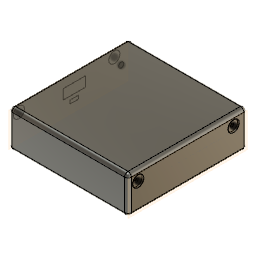
Pedant_lijunchen (Autodesk Fusion 360 design; units mm, degrees)
Autodesk Fusion 360 part; units mm, degrees
sketch "Sketch1" plane through (0, 0, 0) normal (0, 1, 0) x (1, 0, 0) in component "Case"
  line L0 (-35, -10) -> (35, -10)
  line L1 (35, -10) -> (35, 10)
  line L2 (35, 10) -> (-35, 10)
  line L3 (-35, 10) -> (-35, -10)
  dimension "d1" = 70
  dimension "d2" = 20
  dimension "d4" = 35
  dimension "d5" = 10
  constraint horizontal L0
  constraint vertical L1
  constraint horizontal L2
  constraint vertical L3
  measures "d1" distance of L0.start L0.end
  measures "d2" distance of L0.start L2.end
  measures "d4" horizontal distance of origin L0.start
  measures "d5" vertical distance of origin L0.start
extrude "Extrude1" add sketch "Sketch1" along normal blind 70 makes body 1 in component "Case"
shell "Shell1" thickness 2 removed faces 1 at (-11.6667, 23.3333, 10) on bodies 1 in component "Case"
sketch "Sketch2" plane through (-35, 0, 0) normal (-1, 0, 0) x (0, -1, 0) in component "Case"
  line L0 (0, -10) -> (0, 10)
  line L1 (0, 10) -> (-70, 10)
  line L2 (-70, 10) -> (-70, -10)
  line L3 (-70, -10) -> (0, -10)
  circle A0 centre (-66, 0) radius 1.5
  circle A1 centre (-6, 6) radius 3.25
  circle A2 centre (-62, 6) radius 3.25
  line L4 (-45, 5) -> (-32, 5)
  line L5 (-32, 5) -> (-32, -0.8)
  line L6 (-32, -0.8) -> (-45, -0.8)
  line L7 (-45, -0.8) -> (-45, 5)
  line L8 (-41, -2.8) -> (-36, -2.8)
  line L9 (-36, -2.8) -> (-36, -4.8)
  line L10 (-36, -4.8) -> (-41, -4.8)
  line L11 (-41, -4.8) -> (-41, -2.8)
  dimension "d9" = 3
  dimension "d10" = 4
  dimension "d11" = 10
  dimension "d12" = 6.5
  dimension "d14" = 6
  dimension "d15" = 6.5
  dimension "d16" = 8
  dimension "d17" = 4
  dimension "d29" = 13
  dimension "d30" = 5.8
  dimension "d31" = 5
  dimension "d32" = 2
  dimension "d33" = 5
  dimension "d34" = 25
  dimension "d35" = 2
  dimension "d36" = 4
  dimension "d87" = 4
  constraint horizontal L4
  constraint vertical L5
  constraint horizontal L6
  constraint vertical L7
  constraint horizontal L8
  constraint vertical L9
  constraint horizontal L10
  constraint vertical L11
  measures "d9" diameter of A0
  measures "d10" horizontal distance of L1.end A0.centre
  measures "d11" vertical distance of L1.end A0.centre
  measures "d12" diameter of A1
  measures "d14" horizontal distance of L0.end A1.centre
  measures "d15" diameter of A2
  measures "d16" horizontal distance of L1.end A2.centre
  measures "d17" vertical distance of L1.end A2.centre
  measures "d29" distance of L4.start L4.end
  measures "d30" distance of L4.start L6.end
  measures "d31" distance of L8.start L8.end
  measures "d32" distance of L8.start L10.end
  measures "d33" distance of L1 L4.start
  measures "d34" horizontal distance of L1.end L4.start
  measures "d35" vertical distance of L6.end L8.start
  measures "d36" horizontal distance of L6.end L8.start
  measures "d87" vertical distance of L0.end A1.centre
hole "Hole2" at (-35, 6, 6) direction (1, 0, 0) diameter 2 depth 6 tip angle 118 bodies 1 in component "Case"
hole "Hole1" at (-35, 62, 6) direction (1, 0, 0) diameter 2 depth 6 tip angle 118 bodies 1 in component "Case"
extrude "Extrude2" cut sketch "Sketch2" against normal blind 1 contours A1 | A2 bodies 1 in component "Case"
extrude "Extrude3" cut sketch "Sketch2" against normal blind 6 contours A0 | L4 L5 L6 L7 | L8 L9 L10 L11 bodies 1 in component "Case"
sketch "Sketch3" plane through (0, 70, 0) normal (0, 1, 0) x (-1, 0, 0) in component "Case"
  line L0 (35, -10) -> (35, 10)
  line L1 (35, 10) -> (-35, 10)
  line L2 (-35, 10) -> (-35, -10)
  line L3 (-35, -10) -> (35, -10)
  circle A0 centre (31, 0) radius 1.5
  point P0 (35, 10)
  dimension "d39" = 3
  dimension "d40" = 4
  dimension "d41" = 10
  measures "d39" diameter of A0
  measures "d40" horizontal distance of A0.centre P0
  measures "d41" vertical distance of A0.centre P0
extrude "Extrude4" cut sketch "Sketch3" against normal blind 6 contours A0 bodies 1 in component "Case"
sketch "Sketch4" plane through (35, 0, 0) normal (1, 0, 0) x (0, 1, 0) in component "Case"
  line L0 (0, 10) -> (0, -10)
  line L1 (0, -10) -> (70, -10)
  line L2 (70, -10) -> (70, 10)
  line L3 (70, 10) -> (0, 10)
  circle A0 centre (6, 6) radius 3.25
  circle A1 centre (62, 6) radius 3.25
  dimension "d44" = 6.5
  dimension "d45" = 6
  dimension "d46" = 4
  dimension "d47" = 6.5
  dimension "d48" = 8
  dimension "d49" = 4
  measures "d44" diameter of A0
  measures "d45" horizontal distance of L0.start A0.centre
  measures "d46" vertical distance of L0.start A0.centre
  measures "d47" diameter of A1
  measures "d48" horizontal distance of L2.end A1.centre
  measures "d49" vertical distance of L2.end A1.centre
hole "Hole5" at (35, 62, 6) direction (-1, 0, 0) diameter 2 depth 6 tip angle 118 bodies 1 in component "Case"
hole "Hole4" at (35, 6, 6) direction (-1, 0, 0) diameter 2 depth 6 tip angle 118 bodies 1 in component "Case"
extrude "Extrude5" cut sketch "Sketch4" against normal blind 1 contours A0 | A1 bodies 1 in component "Case"
fillet "Fillet1" radius 2 8 edges at (35, 0, 0) (0, 0, -10) (-35, 0, 0) (35, 70, 0) (0, 70, -10) (-35, 70, 0) (-35, 35, -10) (35, 35, -10) on bodies 1 in component "Case"
sketch "Sketch1 (2)" plane through (0, 0, 10) normal (0, 0, 1) x (-1, 0, 0) in component "Top"
  arc A0 (-33, 0) -> (-35, -2) centre (-33, -2) ccw
  line L0 (-35, -2) -> (-35, -68)
  arc A1 (-35, -68) -> (-33, -70) centre (-33, -68) ccw
  line L1 (-33, -70) -> (33, -70)
  arc A2 (33, -70) -> (35, -68) centre (33, -68) ccw
  line L2 (35, -68) -> (35, -2)
  arc A3 (35, -2) -> (33, 0) centre (33, -2) ccw
  line L3 (33, 0) -> (-33, 0)
  line L4 (33, -2) -> (33, -68)
  line L5 (33, -68) -> (-33, -68)
  line L6 (-33, -68) -> (-33, -2)
  line L7 (-33, -2) -> (33, -2)
  line L8 (33, -2) -> (-33, -2)
  line L9 (-33, -2) -> (-33, -68)
  line L10 (-33, -68) -> (33, -68)
  line L11 (33, -68) -> (33, -2)
extrude "Extrude1'" add sketch "Sketch1 (2)" along normal blind 2 separate body contours A0 L0 A1 L1 A2 L2 A3 L3 | L4 L5 L6 L7 L8 L9 L10 L11 makes body 2 in component "Top"
sketch "Sketch2 (2)" plane through (0, 0, 10) normal (0, 0, -1) x (1, 0, 0) in component "Top"
  line L0 (33, 0) -> (-33, 0)
  arc A0 (-33, 0) -> (-35, -2) centre (-33, -2) ccw
  line L1 (-35, -2) -> (-35, -68)
  arc A1 (-35, -68) -> (-33, -70) centre (-33, -68) ccw
  line L2 (-33, -70) -> (33, -70)
  arc A2 (33, -70) -> (35, -68) centre (33, -68) ccw
  line L3 (35, -68) -> (35, -2)
  arc A3 (35, -2) -> (33, 0) centre (33, -2) ccw
  line L4 (-33, -3) -> (-27, -3)
  line L5 (-27, -3) -> (-27, -9)
  line L6 (-27, -9) -> (-33, -9)
  line L7 (-33, -9) -> (-33, -3)
  line L8 (27, -3) -> (33, -3)
  line L9 (33, -3) -> (33, -9)
  line L10 (33, -9) -> (27, -9)
  line L11 (27, -9) -> (27, -3)
  line L12 (-33, -59) -> (-27, -59)
  line L13 (-27, -59) -> (-27, -65)
  line L14 (-27, -65) -> (-33, -65)
  line L15 (-33, -65) -> (-33, -59)
  line L16 (33, -62) -> (33, -68)
  line L17 (33, -68) -> (27, -68)
  line L18 (33, -65) -> (27, -65)
  line L19 (27, -65) -> (27, -59)
  line L20 (27, -59) -> (33, -59)
  line L21 (33, -59) -> (33, -65)
  dimension "d61" = 6
  dimension "d62" = 6
  dimension "d63" = 6
  dimension "d64" = 6
  dimension "d65" = 6
  dimension "d66" = 6
  dimension "d69" = 2
  dimension "d71" = 2
  dimension "d72" = 2
  dimension "d73" = 3
  dimension "d75" = 3
  dimension "d78" = 5
  dimension "d82" = 6
  dimension "d83" = 5
  dimension "d84" = 2
  constraint horizontal L4
  constraint vertical L5
  constraint horizontal L6
  constraint vertical L7
  constraint horizontal L8
  constraint vertical L9
  constraint horizontal L10
  constraint vertical L11
  constraint horizontal L12
  constraint vertical L13
  constraint horizontal L14
  constraint vertical L15
  constraint vertical L16
  constraint horizontal L17
  constraint horizontal L18
  constraint vertical L19
  constraint horizontal L20
  constraint vertical L21
  measures "d61" distance of L4.start L4.end
  measures "d62" distance of L4.start L6.end
  measures "d63" distance of L8.start L8.end
  measures "d64" distance of L8.start L10.end
  measures "d65" distance of L12.start L12.end
  measures "d66" distance of L12.start L14.end
  measures "d69" horizontal distance of L3.end L9.end
  measures "d71" horizontal distance of L1.end L14.end
  measures "d72" horizontal distance of A0.end L4.start
  measures "d73" distance of L0.end L4.start
  measures "d75" distance of L0 L8.end
  measures "d78" distance of A1.end L14.end
  measures "d82" distance of L18.start L20.end
  measures "d83" vertical distance of L2.end L18.start
  measures "d84" horizontal distance of A2.end L18.start
extrude "Extrude2'" add sketch "Sketch2 (2)" along normal blind 8 contours L4 L5 L6 L7 | L8 L9 L10 L11 | L12 L13 L14 L15 | L16 L18 L19 L20 L21 bodies 2 in component "Top"
hole "Hole1'" at (-33, 62, 6) direction (1, 0, 0) diameter 2 depth 6 tip angle 118 bodies 2 in component "Top"
hole "Hole2'" at (-33, 6, 6) direction (1, 0, 0) diameter 2 depth 6 tip angle 118 bodies 2 in component "Top"
hole "Hole3" at (33, 6, 6) direction (-1, 0, 0) diameter 2 depth 6 tip angle 118 bodies 2 in component "Top"
hole "Hole4'" at (33, 62, 6) direction (-1, 0, 0) diameter 2 depth 6 tip angle 118 bodies 2 in component "Top"
fillet "Fillet1'" radius 2 8 edges at (0, 70, 12) (-34.4142, 69.4142, 12) (-35, 35, 12) (-34.4142, 0.5858, 12) (0, 0, 12) (34.4142, 0.5858, 12) (35, 35, 12) (34.4142, 69.4142, 12) on bodies 2 in component "Top"
component "Case" placed x (1, 0, 0) y (0, 1, 0) z (0, 0, 1) at (0, 0, 0)
component "Top" placed x (1, 0, 0) y (0, 1, 0) z (0, 0, 1) at (0, 0, 0)
